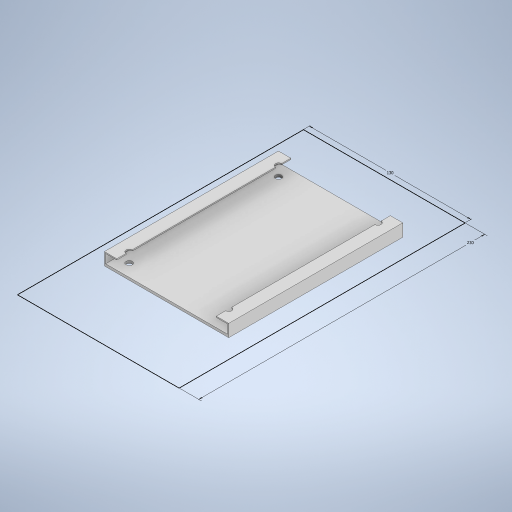
# Autodesk Inventor part: Pieza3
Saved by Autodesk Inventor 2024 (Build 280153000, 153)
## iProperties
Created: 2023-10-22
Part Number: Pieza3
Material: Genérico
Document SubType Name: Modeling
Designer: jhonc
Density: 1 g/cm^3
Appearance: Valor por defecto
Author: jhonc
Autodesk Inventor part; units mm, degrees
ref_plane "YZ Plane" through (0, 0, 0) normal (1, 0, 0) x (0, 1, 0)
ref_plane "XZ Plane" through (0, 0, 0) normal (0, 1, 0) x (-1, 0, 0)
ref_plane "XY Plane" through (0, 0, 0) normal (0, 0, 1) x (1, 0, 0)
sketch "Boceto1" plane through (0, 0, 0) normal (0, 1, 0) x (-1, 0, 0)
  line L0 (0, 0) -> (130, 0)
  line L1 (130, 0) -> (130, -230)
  line L2 (130, -230) -> (0, -230)
  line L3 (0, -230) -> (0, 0)
  dimension "d0" = 130
  dimension "d1" = 230
  constraints: 8 end point, 2 parallel, 1 horizontal, 1 perpendicular
  measures "d0" distance of L1.end L2.end
  measures "d1" distance of L2.end L0.start
extrude "Extrusión1" add sketch "Boceto1" along normal blind 3
sketch "Boceto2" plane through (0, 3, 0) normal (0, 1, 0) x (1, 0, 0)
  line L0 (0, 230) -> (-130, 230) projected
  line L1 (0, 0) -> (-130, 0)
  line L2 (-130, 0) -> (-130, 230)
  line L3 (-130, 230) -> (0, 230)
  line L4 (0, 230) -> (0, 0)
  line L5 (-127, 227) -> (-127, 3)
  line L6 (-127, 3) -> (-3, 3)
  line L7 (-3, 3) -> (-3, 227)
  line L8 (-3, 227) -> (-127, 227)
  dimension "d4" = 3
  constraints: 16 end point, 4 parallel, 2 perpendicular, 1 horizontal, 3 other
  measures "d4" distance between parallel lines of L2 L5
extrude "Extrusión2" add sketch "Boceto2" along normal blind 60
sketch "Boceto3" plane through (-127, 3, -3) normal (1, 0, 0) x (0, 0, -1)
  line L0 (224, 0) -> (224, 60) projected
  line L1 (0, 60) -> (224, 60)
  line L2 (224, 60) -> (224, 59)
  line L3 (224, 59) -> (0, 59)
  line L4 (0, 59) -> (0, 60)
  point P0 (-3, -3)
  dimension "d7" = 1
  constraints: 8 end point, 2 parallel, 1 horizontal, 1 perpendicular, 1 point on line
  measures "d7" distance between parallel lines of L3 L1
extrude "Extrusión3" add sketch "Boceto3" along normal blind 10
sketch "Boceto4" plane through (-117, 3, -3) normal (1, 0, 0) x (0, 0, -1)
  line L0 (0, 59) -> (224, 59) projected
  line L1 (0, 60) -> (10, 60)
  line L2 (10, 60) -> (10, 59)
  line L3 (10, 59) -> (0, 59)
  line L4 (0, 59) -> (0, 60)
  line L5 (224, 60) -> (214, 60)
  line L6 (214, 60) -> (214, 59)
  line L7 (214, 59) -> (224, 59)
  line L8 (224, 59) -> (224, 60)
  point P0 (-3, -3)
  dimension "d10" = 10
  dimension "d11" = 10
  constraints: 16 end point, 4 parallel, 3 point on line, 2 horizontal, 2 perpendicular
  measures "d10" distance of L2.end L3.end
  measures "d11" distance of L7.end L6.end
extrude "Extrusión4" add sketch "Boceto4" along normal blind 115.25
sketch "Boceto5" plane through (-117, 63, -217) normal (0, 0, 1) x (1, 0, 0)
  line L0 (114, -1) -> (104, -1)
  line L1 (104, -1) -> (104, 0)
  line L2 (104, 0) -> (114, 0)
  line L3 (114, 0) -> (114, -1)
  line L4 (0, 0) -> (114, 0) projected
  line L5 (0, -1) -> (114, -1) projected
  point P0 (117, -63)
  dimension "d14" = 10
  dimension "d15" = 0
  dimension "d16" = 0
  constraints: 8 end point, 2 parallel, 1 horizontal, 1 perpendicular
  measures "d14" distance of L1.end L2.end
  measures "d15" distance between parallel lines of L4 L2
  measures "d16" distance between parallel lines of L5 L0
extrude "Extrusión5" add sketch "Boceto5" along normal blind 211.5
sketch "Boceto6" plane through (0, 63, 0) normal (0, 1, 0) x (1, 0, 0)
  circle A0 centre (-10, 220) radius 1.5
  circle A1 centre (-120, 220) radius 1.5
  circle A2 centre (-10, 10) radius 1.5
  circle A3 centre (-120, 10) radius 1.5
  line L0 (-130, 0) -> (0, 0) projected
  line L1 (0, 0) -> (0, 230) projected
  line L2 (-130, 230) -> (-130, 0) projected
  line L3 (0, 230) -> (-130, 230) projected
  dimension "d19" = 3
  dimension "d20" = 3
  dimension "d21" = 3
  dimension "d22" = 3
  dimension "d23" = 10
  dimension "d24" = 10
  dimension "d25" = 10
  dimension "d26" = 10
  dimension "d27" = 10
  dimension "d28" = 10
  dimension "d29" = 10
  dimension "d30" = 10
  constraints: 4 centre point
  measures "d19" diameter of A0
  measures "d20" diameter of A1
  measures "d21" diameter of A2
  measures "d22" diameter of A3
  measures "d23" distance from line of L0 A2.centre
  measures "d24" distance from line of L1 A2.centre
  measures "d25" distance from line of L2 A3.centre
  measures "d26" distance from line of L0 A3.centre
  measures "d27" distance from line of L1 A0.centre
  measures "d28" distance from line of L3 A0.centre
  measures "d29" distance from line of L3 A1.centre
  measures "d30" distance from line of L2 A1.centre
extrude "Extrusión6" cut sketch "Boceto6" against normal blind 211.5 contours A0 | A1 | A2 | A3
sketch "Boceto7" plane through (0, 0, 0) normal (0, -1, 0) x (1, 0, 0)
  circle A0 centre (-25, -205) radius 4
  circle A1 centre (-105, -205) radius 4
  circle A2 centre (-25, -25) radius 4
  circle A3 centre (-105, -25) radius 4
  line L0 (0, 0) -> (0, -230) projected
  line L1 (0, -230) -> (-130, -230) projected
  line L2 (-130, -230) -> (-130, 0) projected
  line L3 (-130, 0) -> (0, 0) projected
  dimension "d33" = 8
  dimension "d34" = 8
  dimension "d35" = 8
  dimension "d36" = 8
  dimension "d37" = 25
  dimension "d38" = 25
  dimension "d39" = 25
  dimension "d40" = 25
  dimension "d41" = 25
  dimension "d42" = 25
  dimension "d43" = 25
  dimension "d44" = 25
  constraints: 4 centre point
  measures "d33" diameter of A0
  measures "d34" diameter of A1
  measures "d35" diameter of A2
  measures "d36" diameter of A3
  measures "d37" distance from line of L0 A0.centre
  measures "d38" distance from line of L1 A0.centre
  measures "d39" distance from line of L2 A1.centre
  measures "d40" distance from line of L1 A1.centre
  measures "d41" distance from line of L3 A2.centre
  measures "d42" distance from line of L0 A2.centre
  measures "d43" distance from line of L3 A3.centre
  measures "d44" distance from line of L2 A3.centre
extrude "Extrusión7" cut sketch "Boceto7" against normal blind 10 contours A0 | A1 | A2 | A3
sketch "Boceto8" plane through (0, 0, 0) normal (0, -1, 0) x (1, 0, 0)
  line L0 (-30, -35) -> (-100, -35)
  line L1 (-100, -35) -> (-100, -45)
  line L2 (-100, -45) -> (-30, -45)
  line L3 (-30, -45) -> (-30, -35)
  line L4 (-130, 0) -> (0, 0) projected
  line L5 (0, 0) -> (0, -230) projected
  line L6 (-130, -230) -> (-130, 0) projected
  circle A0 centre (-35, -40) radius 2.5
  circle A1 centre (-95, -40) radius 2.5
  point P0 (-30, -40)
  dimension "d47" = 70
  dimension "d48" = 10
  dimension "d49" = 35
  dimension "d50" = 30
  dimension "d51" = 30
  dimension "d52" = 5
  dimension "d53" = 5
  dimension "d54" = 5
  dimension "d55" = 5
  dimension "d56" = 5
  dimension "d57" = 5
  constraints: 8 end point, 2 centre point, 2 parallel, 1 horizontal, 1 midpoint, 1 perpendicular
  measures "d47" distance of L2.end L1.end
  measures "d48" distance between parallel lines of L2 L0
  measures "d49" distance between parallel lines of L4 L0
  measures "d50" distance between parallel lines of L5 L3
  measures "d51" distance between parallel lines of L6 L1
  measures "d52" diameter of A0
  measures "d53" diameter of A1
  measures "d54" distance of point (-30, -40) A0.centre
  measures "d55" distance from line of L1 A1.centre
  measures "d56" distance from line of L2 A1.centre
  measures "d57" distance from line of L2 A0.centre
extrude "Extrusión8" cut sketch "Boceto8" against normal blind 10 contours A0 | A1
sketch "Boceto9" plane through (0, 0, 0) normal (0, -1, 0) x (1, 0, 0)
  line L0 (-20, -190) -> (-110, -190)
  line L1 (-110, -190) -> (-110, -60)
  line L2 (-110, -60) -> (-20, -60)
  line L3 (-20, -60) -> (-20, -190)
  line L4 (0, 0) -> (0, -230) projected
  line L5 (-130, -230) -> (-130, 0) projected
  line L6 (-130, 0) -> (0, 0) projected
  circle A0 centre (-25, -185) radius 2.5
  circle A1 centre (-25, -65) radius 2.5
  circle A2 centre (-105, -65) radius 2.5
  circle A3 centre (-105, -185) radius 2.5
  dimension "d60" = 90
  dimension "d61" = 130
  dimension "d62" = 20
  dimension "d63" = 20
  dimension "d64" = 60
  dimension "d65" = 5
  dimension "d66" = 5
  dimension "d67" = 5
  dimension "d68" = 5
  dimension "d69" = 5
  dimension "d70" = 5
  dimension "d71" = 5
  dimension "d72" = 5
  dimension "d73" = 5
  dimension "d74" = 5
  dimension "d75" = 5
  dimension "d76" = 5
  constraints: 8 end point, 4 centre point, 2 parallel, 1 horizontal, 1 perpendicular
  measures "d60" distance of L0.start L0.end
  measures "d61" distance of L0.end L1.end
  measures "d62" distance between parallel lines of L4 L3
  measures "d63" distance between parallel lines of L5 L1
  measures "d64" distance between parallel lines of L6 L2
  measures "d65" diameter of A0
  measures "d66" diameter of A1
  measures "d67" diameter of A2
  measures "d68" diameter of A3
  measures "d69" distance from line of L3 A0.centre
  measures "d70" distance from line of L0 A0.centre
  measures "d71" distance from line of L1 A3.centre
  measures "d72" distance from line of L0 A3.centre
  measures "d73" distance from line of L3 A1.centre
  measures "d74" distance from line of L2 A1.centre
  measures "d75" distance from line of L1 A2.centre
  measures "d76" distance from line of L2 A2.centre
extrude "Extrusión9" cut sketch "Boceto9" against normal blind 10 contours A0 | A1 | A2 | A3
sketch "Boceto11" plane through (0, 63, 0) normal (0, 1, 0) x (1, 0, 0)
  line L0 (-230.0178, 308.5075) -> (121.3875, 308.5075)
  line L1 (121.3875, 308.5075) -> (121.3875, -22.7652)
  line L2 (121.3875, -22.7652) -> (-230.0178, -22.7652)
  line L3 (-230.0178, -22.7652) -> (-230.0178, 308.5075)
  point P0 (0, 0)
  constraints: 8 end point, 2 parallel, 1 horizontal, 1 perpendicular
extrude "Extrusión10" cut sketch "Boceto11" against normal blind 61
sketch "Boceto12" plane through (0, 2, 0) normal (0, 1, 0) x (1, 0, 0)
  circle A0 centre (-105, 185) radius 2.5 projected
  circle A1 centre (-25, 65) radius 2.5 projected
  line L0 (-105, 185) -> (-25, 185)
  line L1 (-25, 185) -> (-25, 65)
  line L2 (-25, 65) -> (-105, 65)
  line L3 (-105, 65) -> (-105, 185)
  line L4 (-158.8037, 262.2681) -> (33.433, 262.2681)
  line L5 (33.433, 262.2681) -> (33.433, -27.1386)
  line L6 (33.433, -27.1386) -> (-158.8037, -27.1386)
  line L7 (-158.8037, -27.1386) -> (-158.8037, 262.2681)
  line L8 (-15, 55) -> (-15, 195)
  line L9 (-15, 195) -> (-115, 195)
  line L10 (-115, 195) -> (-115, 55)
  line L11 (-115, 55) -> (-15, 55)
  circle A2 centre (-105, 185) radius 2.5
  circle A3 centre (-25, 185) radius 2.5 projected
  circle A4 centre (-25, 185) radius 2.5
  circle A5 centre (-105, 65) radius 2.5 projected
  circle A6 centre (-105, 65) radius 2.5
  circle A7 centre (-25, 65) radius 2.5
  point P0 (0, 0)
  dimension "d81" = 10
  constraints: 24 end point, 6 parallel, 4 centre point, 4 coincident, 3 perpendicular, 2 concentric, 2 horizontal, 3 other
  measures "d81" distance between parallel lines of L1 L8
extrude "Extrusión11" cut sketch "Boceto12" against normal blind 61 contours L4 L5 L6 L7
sketch "Boceto13" plane through (-15, 2, -195) normal (0, 0, -1) x (-1, 0, 0)
  line L0 (100, 0) -> (100, -2) projected
  line L1 (100, -2) -> (99, -2)
  line L2 (99, -2) -> (99, 8)
  line L3 (99, 8) -> (100, 8)
  line L4 (100, 8) -> (100, -2)
  line L5 (0, -2) -> (1, -2)
  line L6 (1, -2) -> (1, 8)
  line L7 (1, 8) -> (0, 8)
  line L8 (0, 8) -> (0, -2)
  line L9 (0, 0) -> (0, -2) projected
  line L10 (100, 8) -> (0, 8)
  line L11 (0, 8) -> (0, 7.1109)
  line L12 (0, 7.1109) -> (100, 7.1109)
  line L13 (100, 7.1109) -> (100, 8)
  line L14 (90, 7.1109) -> (10, 7.1109)
  line L15 (10, 7.1109) -> (10, 8)
  line L16 (10, 8) -> (90, 8)
  line L17 (90, 8) -> (90, 7.1109)
  line L18 (100, 0) -> (0, 0)
  line L19 (0, 0) -> (0, 8)
  line L20 (0, 8) -> (100, 8)
  line L21 (100, 8) -> (100, 0)
  point P0 (-15, -2)
  point P1 (0, -1)
  point P2 (90, 7.5554)
  point P3 (10, 7.5554)
  point P4 (99, 0)
  point P5 (99, 7.1109)
  point P6 (10, 7.1109)
  point P7 (1, 8)
  point P8 (1, 0)
  point P9 (1, 7.1109)
  dimension "d84" = 1
  dimension "d85" = 1
  dimension "d86" = 0
  dimension "d87" = 10
  dimension "d88" = 10
  dimension "d89" = 100
  dimension "d90" = 10
  dimension "d91" = 10
  constraints: 40 end point, 10 parallel, 5 horizontal, 5 perpendicular, 3 midpoint, 3 point on line
  measures "d84" distance of L2.end L3.end
  measures "d85" distance from line of point (0, -1) L6
  measures "d86" distance between parallel lines of L9 L8
  measures "d87" distance of L3.end L0.end
  measures "d88" distance of L7.end L5.start
  measures "d89" distance of L12.end L11.end
  measures "d90" distance from line of point (90, 7.555) L4
  measures "d91" distance from line of L8 point (10, 7.555)
extrude "Extrusión12" add sketch "Boceto13" against normal blind 140 contours L18 L2 L12 L4 | L12 L2 L3 L4 | L12 L17 L10 L2 | L18 L8 L12 L6 | L12 L8 L7 L6 | L6 L10 L15 L12
sketch "Boceto14" plane through (0, 0, 0) normal (0, -1, 0) x (1, 0, 0)
  circle A0 centre (-25, -65) radius 2.5 projected
  circle A1 centre (-25, -65) radius 2.5
  line L0 (-25, -195) -> (-25, -55) projected
  circle A2 centre (-25, -185.0047) radius 2.4975
  line L1 (-105, -195) -> (-105, -55) projected
  circle A3 centre (-105, -185.0047) radius 2.4775
  circle A4 centre (-105, -65) radius 2.5 projected
  circle A5 centre (-105, -65) radius 2.5
  point P0 (0, 0)
  constraints: 4 centre point, 2 coincident, 2 point on line
extrude "Extrusión13" cut sketch "Boceto14" against normal blind 140
